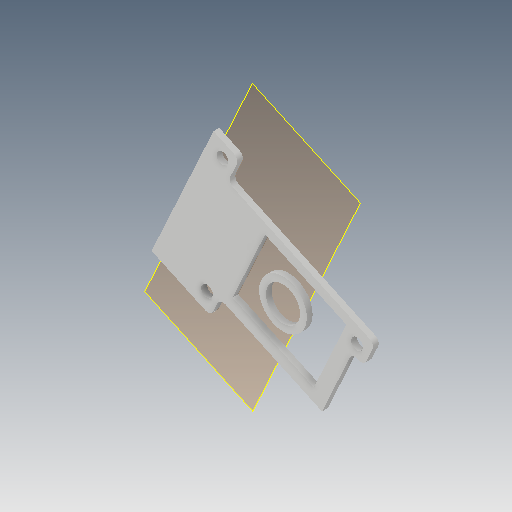
# Autodesk Inventor part: 00_KES400_Bluray_Lens
Saved by Autodesk Inventor 2019 (Build 230136000, 136)
## iProperties
Created: 2018-10-09
Part Number: 00_KES400_Bluray_Lens
Material: Generic
Document SubType Name: Modeling
Designer: diederichbenedict
Density: 1 g/cm^3
Appearance: Default
Author: diederichbenedict
Autodesk Inventor part; units mm, degrees
ref_plane "YZ Plane" through (0, 0, 0) normal (1, 0, 0) x (0, 1, 0)
ref_plane "XZ Plane" through (0, 0, 0) normal (0, 1, 0) x (-1, 0, 0)
ref_plane "XY Plane" through (0, 0, 0) normal (0, 0, 1) x (1, 0, 0)
ref_plane "Work Plane1" through (7.2162, 6.7561, 0) normal (0, 0, 1) x (-0.4175, -0.9087, 0)
sketch "Sketch1" plane through (7.2162, 6.7561, 0) normal (0, 0, 1) x (-0.4175, -0.9087, 0)
  circle A0 centre (9.1366, 15.6864) radius 1
  circle A1 centre (24.6366, -5.8136) radius 1
  circle A2 centre (4.1366, -12.3136) radius 1
  line L0 (21.6366, -2.3136) -> (8.1366, -2.3136)
  line L1 (8.1366, -2.3136) -> (8.1366, 13.1864)
  line L2 (8.1366, 13.1864) -> (21.6366, 13.1864)
  line L3 (21.6366, 13.1864) -> (21.6366, -2.3136)
  line L4 (11.1138, 15.6864) -> (23.6484, 15.6864)
  line L5 (23.6484, 15.6864) -> (23.6484, -3.7858)
  line L6 (23.6484, -3.7858) -> (27.5108, -3.7858)
  line L7 (27.5108, -3.7858) -> (27.5108, -8.9631)
  line L8 (27.5108, -8.9631) -> (27.5108, -15.0789)
  line L9 (27.5108, -15.0789) -> (1.8108, -15.0789)
  line L10 (1.8108, -15.0789) -> (1.8108, -10.169)
  line L11 (1.8108, -10.169) -> (6.5484, -10.169)
  line L12 (6.5484, -10.169) -> (6.5484, 17.9211)
  line L13 (6.5484, 17.9211) -> (11.1138, 17.9211)
  line L14 (11.1138, 17.9211) -> (11.1138, 15.6864)
  point P0 (9.1519, -3.7364)
  dimension "d0" = 2
  dimension "d1" = 2
  dimension "d2" = 2
  dimension "d3" = 28
  dimension "d5" = 15.5
  dimension "d6" = 5
  dimension "d7" = 21.5
  dimension "d8" = 20.5
  dimension "d9" = 2.5
  dimension "d10" = 1
  dimension "d11" = 3.5
  dimension "d12" = 3
  dimension "d13" = 33
  dimension "d14" = 25.7
  dimension "d15" = 17.1
  constraints: 30 end point, 10 perpendicular, 3 centre point, 2 horizontal, 2 parallel, 1 point on line
  measures "d0" diameter of A0
  measures "d1" diameter of A1
  measures "d2" diameter of A2
  measures "d3" vertical distance of A0.centre A2.centre
  measures "d5" horizontal distance of A0.centre A1.centre
  measures "d6" horizontal distance of A2.centre A0.centre
  measures "d7" vertical distance of A0.centre A1.centre
  measures "d8" horizontal distance of A2.centre A1.centre
  measures "d9" distance from line of A0.centre L2
  measures "d10" distance from line of L1 A0.centre
  measures "d11" distance from line of L0 A1.centre
  measures "d12" distance from line of A1.centre L3
  measures "d13" distance between parallel lines of L13 L9
  measures "d14" distance between parallel lines of L10 L7
  measures "d15" distance between parallel lines of L5 L12
extrude "Extrusion1" add sketch "Sketch1" along normal blind 1
fillet "Fillet1" radius 1 7 edges at (20.7666, -6.6764, 0.5) (18.8605, -10.8249, 0.5) (16.83, -9.8919, 0.5) (-6.0973, -13.1521, 0.5) (-7.7098, -16.6617, 0.5) (-2.7802, 9.3562, 0.5) (-4.7582, 5.0513, 0.5)
sketch "Sketch2" plane through (7.2162, 6.7561, 1) normal (0, 0, 1) x (-0.4175, -0.9087, 0)
  circle A0 centre (13.5484, 4.6864) radius 4.149
  circle A1 centre (13.5484, 4.6864) radius 2.9629
  arc A2 (2.8108, -10.169) -> (1.8108, -11.169) centre (2.8108, -11.169) ccw projected
  line L0 (1.8108, -11.169) -> (1.8108, -15.0789) projected
  line L1 (1.8108, -15.0789) -> (27.5108, -15.0789) projected
  line L2 (27.5108, -15.0789) -> (27.5108, -4.7858) projected
  arc A3 (27.5108, -4.7858) -> (26.5108, -3.7858) centre (26.5108, -4.7858) ccw projected
  line L3 (26.5108, -3.7858) -> (24.6484, -3.7858) projected
  arc A4 (23.6484, -2.7858) -> (24.6484, -3.7858) centre (24.6484, -2.7858) ccw projected
  line L4 (23.6484, -2.7858) -> (23.6484, 15.6864) projected
  line L5 (23.6484, 15.6864) -> (12.1138, 15.6864) projected
  arc A5 (11.1138, 16.6864) -> (12.1138, 15.6864) centre (12.1138, 16.6864) ccw projected
  line L6 (11.1138, 16.6864) -> (11.1138, 16.9211) projected
  arc A6 (11.1138, 16.9211) -> (10.1138, 17.9211) centre (10.1138, 16.9211) ccw projected
  line L7 (10.1138, 17.9211) -> (7.5484, 17.9211) projected
  arc A7 (7.5484, 17.9211) -> (6.5484, 16.9211) centre (7.5484, 16.9211) ccw projected
  line L8 (6.5484, 16.9211) -> (6.5484, -9.169) projected
  arc A8 (5.5484, -10.169) -> (6.5484, -9.169) centre (5.5484, -9.169) ccw projected
  line L9 (5.5484, -10.169) -> (2.8108, -10.169) projected
  line L10 (8.1366, -2.3136) -> (8.1366, 13.1864) projected
  line L11 (8.1366, 13.1864) -> (21.6366, 13.1864) projected
  line L12 (21.6366, 13.1864) -> (21.6366, -2.3136) projected
  line L13 (21.6366, -2.3136) -> (8.1366, -2.3136) projected
  circle A9 centre (4.1366, -12.3136) radius 1 projected
  circle A10 centre (24.6366, -5.8136) radius 1 projected
  circle A11 centre (9.1366, 15.6864) radius 1 projected
  point P0 (9.1519, -3.7364)
  dimension "d19" = 11
  dimension "d20" = 7
  constraints: 2 centre point, 1 coincident
  measures "d19" vertical distance of A0.centre A11.centre
  measures "d20" distance from line of A0.centre L8
extrude "Extrusion2" add sketch "Sketch2" along normal blind 1 contours A0
body "Solid1"
